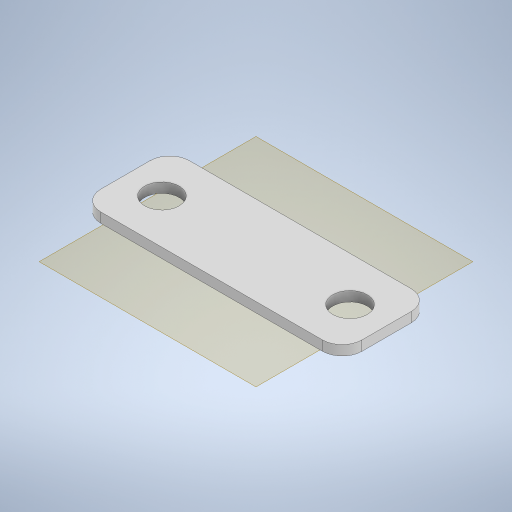
# Autodesk Inventor part: prent1
Saved by Autodesk Inventor 2023 (Build 270158000, 158)
## iProperties
Created: 2023-01-05
Part Number: prent1
Material: Ogólny
Document SubType Name: Modeling
Designer: User
Density: 1 g/cm^3
Appearance: Domyślna
Author: User
Autodesk Inventor part; units mm, degrees
ref_plane "YZ Plane" through (0, 0, 0) normal (1, 0, 0) x (0, 1, 0)
ref_plane "XZ Plane" through (0, 0, 0) normal (0, 1, 0) x (-1, 0, 0)
ref_plane "XY Plane" through (0, 0, 0) normal (0, 0, 1) x (1, 0, 0)
ref_plane "Płaszczyzna konstrukcyjna1" through (0, 0.1, -1.5872) normal (0, 1, 0) x (1, 0, 0)
sketch "Szkic3" plane through (0, 0.1, -1.5872) normal (0, 1, 0) x (1, 0, 0)
  line L0 (6, 4.5) -> (-6, 4.5)
  line L1 (-6, 4.5) -> (-6, -4.5)
  line L2 (-6, -4.5) -> (6, -4.5)
  line L3 (6, -4.5) -> (6, 4.5)
  line L4 (9.543, 0) -> (-12.3472, 0)
  line L5 (0, 10.0787) -> (0, -13.253)
  line L6 (6, 4.5) -> (11.25, 4.5)
  line L7 (13.25, 2.5) -> (13.25, -2.5)
  line L8 (11.25, -4.5) -> (6, -4.5)
  line L9 (6, -4.5) -> (6, 4.5)
  arc A0 (13.25, 2.5) -> (11.25, 4.5) centre (11.25, 2.5) ccw
  arc A1 (11.25, -4.5) -> (13.25, -2.5) centre (11.25, -2.5) ccw
  line L10 (-13.25, 2.5) -> (-13.25, -2.5)
  arc A2 (-11.25, 4.5) -> (-13.25, 2.5) centre (-11.25, 2.5) ccw
  line L11 (-6, 4.5) -> (-11.25, 4.5)
  arc A3 (-13.25, -2.5) -> (-11.25, -4.5) centre (-11.25, -2.5) ccw
  line L12 (-11.25, -4.5) -> (-6, -4.5)
  line L13 (-13.25, 0.45) -> (-9, 0.45)
  circle A4 centre (9.543, 0) radius 1.75
  circle A5 centre (-9.543, 0) radius 1.75
  point P0 (0, 0)
  point P1 (13.25, 4.5)
  dimension "d26" = 12
  dimension "d25" = 9
  dimension "d24" = 4.5
  dimension "d23" = 6
  dimension "d22" = 7.25
  dimension "d20" = 2
  dimension "d19" = 4.25
  dimension "d18" = 4.05
  dimension "d16" = 19.086
  dimension "d21" = 3.707
  dimension "d17" = 3.5
  dimension "d15" = 3.5
  constraints: 28 end point, 8 point on circle, 7 symmetric about line, 6 centre point, 4 horizontal, 4 parallel, 4 point on line, 4 tangent, 3 perpendicular, 2 vertical, 1 coincident, 1 equal radius, 2 other
  measures "d26" distance of L0.start L0.end
  measures "d25" distance of L2.end L0.start
  measures "d24" distance between parallel lines of L4 L0
  measures "d23" distance between parallel lines of L5 L3
  measures "d22" distance of L0.start point (13.25, 4.5)
  measures "d20" radius of A0
  measures "d19" distance of L13.start L13.end
  measures "d18" distance from line of L11 L13.end
  measures "d16" distance of A5.centre L4.start
  measures "d21" distance from line of L4.start L7
  measures "d17" diameter of A4
  measures "d15" diameter of A5
extrude "Wyciągnięcie proste3" add sketch "Szkic3" along normal blind 1 contours L3 L4 L5 L0 | L6 A0 L7 A1 L8 L3 | L5 L4 L1 L0 | L3 L2 L5 L4 | L1 L4 A5 L13 L10 A2 L11 | L5 L2 L1 L4 | L1 L12 A3 L10 L13 A5 L4
